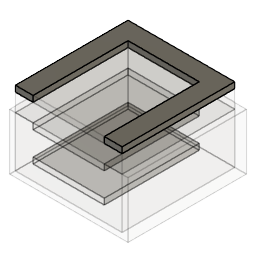
v3 (Autodesk Fusion 360 design; units mm, degrees)
part number: 2026-06-08-14-21-14-896
part number: 2026-06-08-14-24-47-444
part number: 2026-06-08-14-29-35-027
part number: 2026-06-08-14-30-01-795
part number: 2026-06-08-14-32-20-019
part number: 2026-06-08-14-37-08-306
part number: 2026-06-08-14-38-58-466
part number: 2026-06-08-14-44-18-946
part number: 2026-06-08-14-46-16-882
part number: 2026-06-09-12-46-36-713
Autodesk Fusion 360 part; units mm, degrees
sketch "Esquisse1" plane through (0, 0, 0) normal (0, 0, 1) x (1, 0, 0)
  line L0 (0, 0) -> (40, 0)
  line L1 (40, 0) -> (40, 40)
  line L2 (40, 40) -> (0, 40)
  line L3 (0, 40) -> (0, 0)
  dimension "d11" = 40
  dimension "d12" = 40
  constraint horizontal L0
  constraint vertical L1
  constraint horizontal L2
  constraint vertical L3
  constraint coincident L0.start L3.end
  measures "d11" distance of L0.start L0.end
  measures "d12" distance of L0.start L2.end
sketch "Esquisse1 (2)" plane through (0, 0, 2) normal (0, 0, 1) x (-1, 0, 0) in component "Shield"
  line L0 (0, -36) -> (0, 0)
  line L1 (0, 0) -> (-36, 0)
  line L2 (-36, 0) -> (-36, -36)
  line L3 (-36, -36) -> (0, -36)
  line L4 (0, -36) -> (-2, -36)
  line L5 (-2, -36) -> (-2, 4)
  line L6 (-2, 4) -> (0, 4)
  line L7 (0, 4) -> (0, -36)
  line L8 (0, -36) -> (-40, -36)
  line L9 (-40, -36) -> (-40, -34)
  line L10 (-40, -34) -> (0, -34)
  line L11 (0, -34) -> (0, -36)
  line L12 (-40, -36) -> (-38, -36)
  line L13 (-38, -36) -> (-38, 4)
  line L14 (-38, 4) -> (-40, 4)
  line L15 (-40, 4) -> (-40, -36)
  line L16 (-40, 4) -> (0, 4)
  line L17 (0, 4) -> (0, 2)
  line L18 (0, 2) -> (-40, 2)
  line L19 (-40, 2) -> (-40, 4)
  dimension "d15" = 2
  dimension "d16" = 40
  dimension "d17" = 40
  dimension "d18" = 2
  dimension "d19" = 2
  dimension "d20" = 40
  dimension "d21" = 40
  dimension "d22" = 2
  constraint horizontal L4
  constraint vertical L5
  constraint horizontal L6
  constraint vertical L7
  constraint coincident L0.start L3.end
  constraint horizontal L8
  constraint vertical L9
  constraint horizontal L10
  constraint vertical L11
  constraint horizontal L12
  constraint vertical L13
  constraint horizontal L14
  constraint vertical L15
  constraint horizontal L16
  constraint vertical L17
  constraint horizontal L18
  constraint vertical L19
  measures "d15" distance of L0.start L4.end
  measures "d16" distance of L0.start L6.end
  measures "d17" distance of L0.start L8.end
  measures "d18" distance of L0.start L10.end
  measures "d19" distance of L8.end L12.end
  measures "d20" distance of L8.end L14.end
  measures "d21" distance of L14.end L6.end
  measures "d22" distance of L14.end L18.end
sketch "Esquisse2" plane through (0, 0, 2) normal (0, 0, 1) x (-1, 0, 0) in component "Shield"
  line L0 (-36, -2) -> (-34, -2)
  line L1 (-34, -2) -> (-34, -34)
  line L2 (-34, -34) -> (-2, -34)
  line L3 (-2, -34) -> (-2, -2)
  line L4 (-2, -2) -> (0, -2)
  line L5 (0, -2) -> (0, 0)
  line L6 (0, 0) -> (-36, 0)
  line L7 (-36, 0) -> (-36, -2)
sketch "Esquisse1 (3)" plane through (0, 0, 6) normal (0, 0, 1) x (-1, 0, 0) in component "e*"
  line L0 (-36, 0) -> (-36, -2)
  line L1 (-36, -2) -> (-34, -2)
  line L2 (-34, -2) -> (-34, -34)
  line L3 (-34, -34) -> (-2, -34)
  line L4 (-2, -34) -> (-2, -2)
  line L5 (-2, -2) -> (0, -2)
  line L6 (0, -2) -> (0, 0)
  line L7 (0, 0) -> (-36, 0)
  line L8 (-8, -28) -> (-28, -28)
  line L9 (-28, -28) -> (-28, -3.2536)
  line L10 (-28, -3.2536) -> (-8, -3.2536)
  line L11 (-8, -3.2536) -> (-8, -28)
  dimension "d27" = 6
  dimension "d28" = 6
  dimension "d30" = 6
  constraint horizontal L8
  constraint vertical L9
  constraint horizontal L10
  constraint vertical L11
  measures "d27" distance of L4 L11
  measures "d28" distance of L2 L9
  measures "d30" distance of L3 L8
sketch "Esquisse1 (4)" plane through (0, 0, 16) normal (0, 0, 1) x (-1, 0, 0) in component "plaque_haut"
  line L0 (-2, 0) -> (-34, 0)
  line L1 (-34, 0) -> (-34, -34)
  line L2 (-34, -34) -> (-2, -34)
  line L3 (-2, -34) -> (-2, 0)
  line L4 (-6, -30) -> (-30, -30)
  line L5 (-30, -30) -> (-30, 0)
  line L6 (-30, 0) -> (-6, 0)
  line L7 (-6, 0) -> (-6, -30)
  dimension "d39" = 24
  dimension "d40" = 30
  constraint horizontal L4
  constraint vertical L5
  constraint horizontal L6
  constraint vertical L7
  measures "d39" distance of L4.start L4.end
  measures "d40" distance of L4.start L6.end
sketch "Esquisse1 (5)" plane through (0, 0, 18) normal (0, 0, 1) x (-1, 0, 0) in component "Mousse_haute"
  line L0 (0, -36) -> (0, -2)
  line L1 (0, -2) -> (-2, -2)
  line L2 (-2, -2) -> (-2, -34)
  line L3 (-2, -34) -> (-34, -34)
  line L4 (-34, -34) -> (-34, -2)
  line L5 (-34, -2) -> (-36, -2)
  line L6 (-36, -2) -> (-36, -36)
  line L7 (-36, -36) -> (0, -36)
  line L8 (0, -36) -> (-36, -36)
  line L9 (-36, -36) -> (-36, 0)
  line L10 (-36, 0) -> (0, 0)
  line L11 (0, 0) -> (0, -36)
  constraint horizontal L8
  constraint vertical L9
  constraint horizontal L10
  constraint vertical L11
  constraint coincident L0.start L7.end
sketch "Esquisse2 (2)" plane through (0, 0, 0) normal (0, 0, 1) x (1, 0, 0)
  line L0 (0, 0) -> (40, 0)
  line L1 (40, 0) -> (40, 40)
  line L2 (40, 40) -> (0, 40)
  line L3 (0, 40) -> (0, 0)
  dimension "d85" = 40
  dimension "d86" = 40
  constraint horizontal L0
  constraint vertical L1
  constraint horizontal L2
  constraint vertical L3
  constraint coincident L0.start L3.end
  measures "d85" distance of L0.start L0.end
  measures "d86" distance of L0.start L2.end
extrude "Extrusion4" add sketch "Esquisse2 (2)" along normal blind 2 makes body 1 in component "Shield"
sketch "Esquisse3" plane through (0, 0, 2) normal (0, 0, 1) x (-1, 0, 0)
  line L0 (0, -40) -> (0, 0)
  line L1 (0, 0) -> (-40, 0)
  line L2 (-40, 0) -> (-40, -40)
  line L3 (-40, -40) -> (0, -40)
  line L4 (0, -40) -> (-2, -40)
  line L5 (-2, -40) -> (-2, 0)
  line L6 (-2, 0) -> (0, 0)
  line L7 (0, 0) -> (0, -40)
  line L8 (0, -40) -> (-40, -40)
  line L9 (-40, -40) -> (-40, -38)
  line L10 (-40, -38) -> (0, -38)
  line L11 (0, -38) -> (0, -40)
  line L12 (-40, -40) -> (-38, -40)
  line L13 (-38, -40) -> (-38, 0)
  line L14 (-38, 0) -> (-40, 0)
  line L15 (-40, 0) -> (-40, -40)
  dimension "d89" = 2
  dimension "d90" = 40
  dimension "d91" = 40
  dimension "d92" = 2
  dimension "d93" = 2
  dimension "d94" = 40
  constraint horizontal L4
  constraint vertical L5
  constraint horizontal L6
  constraint vertical L7
  constraint coincident L0.start L3.end
  constraint horizontal L8
  constraint vertical L9
  constraint horizontal L10
  constraint vertical L11
  constraint horizontal L12
  constraint vertical L13
  constraint horizontal L14
  constraint vertical L15
  measures "d89" distance of L0.start L4.end
  measures "d90" distance of L0.start L0.end
  measures "d91" distance of L0.start L2.end
  measures "d92" distance of L0.start L10.end
  measures "d93" distance of L2.end L12.end
  measures "d94" distance of L2.end L1.end
extrude "Extrusion15" add sketch "Esquisse3" along normal blind 5 separate body contours L1 L5 L10 L13 makes body 2 in component "Support"
sketch "Esquisse1 (6)" plane through (0, 0, 7) normal (0, 0, 1) x (-1, 0, 0) in component "Plaque bas"
  line L0 (-38, -38) -> (-2, -38)
  line L1 (-2, -38) -> (-2, 0)
  line L2 (-2, 0) -> (-38, 0)
  line L3 (-38, 0) -> (-38, -38)
  line L4 (-8, 0) -> (-32, 0)
  line L5 (-32, 0) -> (-32, -32)
  line L6 (-32, -32) -> (-8, -32)
  line L7 (-8, -32) -> (-8, 0)
  dimension "d100" = 6
  dimension "d101" = 6
  dimension "d102" = 6
  constraint horizontal L4
  constraint vertical L5
  constraint horizontal L6
  constraint vertical L7
  constraint coincident L2 L4.start
  measures "d100" distance of L1 L7
  measures "d101" distance of L3 L5
  measures "d102" distance of L0 L6
extrude "Extrusion16" add sketch "Esquisse1 (6)" along normal blind 2 contours L0 L1 L2 L3 L5 L6 L7 bodies 2 in component "Support"
extrude "Extrusion5" add 1 faces at (16, 21.3333, 7) along direction (0, 0, 1) blind 2 separate body on bodies 2 makes body 3 in component "Plaque bas"
extrude "Extrusion17" add 1 faces at (36, 23.3333, 9) along direction (0, 0, 1) blind 8 on bodies 2 bodies 2 in component "Support"
extrude "Extrusion18" add 1 faces at (16, 21.3333, 9) along direction (0, 0, 1) blind 8 on bodies 3 bodies 2 in component "Support"
sketch "Esquisse2 (3)" plane through (0, 0, 17) normal (0, 0, 1) x (-1, 0, 0) in component "plaque_haut"
  line L0 (-2, 0) -> (-38, 0)
  line L1 (-38, 0) -> (-38, -38)
  line L2 (-38, -38) -> (-2, -38)
  line L3 (-2, -38) -> (-2, 0)
  line L4 (-8, 0) -> (-32, 0)
  line L5 (-32, 0) -> (-32, -32)
  line L6 (-32, -32) -> (-8, -32)
  line L7 (-8, -32) -> (-8, 0)
  point P0 (-32, 0)
  dimension "d111" = 6
  dimension "d112" = 6
  dimension "d113" = 6
  constraint horizontal L4
  constraint vertical L5
  constraint horizontal L6
  constraint vertical L7
  constraint coincident L4 P0
  measures "d111" distance of L2 L6
  measures "d112" distance of L1 L5
  measures "d113" distance of L3 L7
extrude "Extrusion5'" add sketch "Esquisse2 (3)" along normal blind 2 separate body contours L0 L4 L5 L6 L7 makes body 4 in component "plaque_haut"
extrude "Extrusion19" add 1 faces at (14, 12.6667, 17) along direction (0, 0, 1) blind 2 on bodies 2 bodies 2 in component "Support"
copy_body "CopierCollerCorps3" bodies 4 makes body 5 in component "Support"
combine "Combiner2" operation cut target body 2 tool bodies 5 in component "Support"
extrude "Extrusion2" add 1 faces at (16, 21.3333, 19) along direction (0, 0, 1) blind 6 separate body on bodies 4 makes body 6 in component "Mousse_haute"
extrude "Extrusion3" add 1 faces at (36, 23.3333, 19) along direction (0, 0, 1) blind 6 on bodies 2 bodies 6 in component "Mousse_haute"
extrude "Extrusion5''" add 1 faces at (13.3333, 13.3333, 2) along direction (0, 0, 1) blind 17 on bodies 1 bodies 1 in component "Shield"
copy_body "CopierCollerCorps1" bodies 3 makes body 7 in component "Shield"
copy_body "CopierCollerCorps2" bodies 4 7 makes body 8 makes body 9 in component "Shield"
copy_body "CopierCollerCorps3'" bodies 4 makes body 10 in component "Shield"
combine "Combiner1" operation cut target body 1 tool bodies 7 8 9 10 in component "Shield"
sketch "Esquisse1 (7)" plane through (0, 0, 25) normal (0, 0, 1) x (-1, 0, 0) in component "Support"
  line L0 (-2, 0) -> (-38, 0)
  line L1 (-38, 0) -> (-38, -38)
  line L2 (-38, -38) -> (-2, -38)
  line L3 (-2, -38) -> (-2, 0)
  line L4 (-8, 0) -> (-32, 0)
  line L5 (-32, 0) -> (-32, -32)
  line L6 (-32, -32) -> (-8, -32)
  line L7 (-8, -32) -> (-8, 0)
  dimension "d124" = 6
  dimension "d125" = 6
  dimension "d126" = 6
  constraint horizontal L4
  constraint vertical L5
  constraint horizontal L6
  constraint vertical L7
  constraint coincident L0 L4.start
  measures "d124" distance of L1 L5
  measures "d125" distance of L3 L7
  measures "d126" distance of L2 L6
extrude "Extrusion2'" add sketch "Esquisse1 (7)" along normal blind 2 separate body contours L0 L4 L5 L6 L7 makes body 11 in component "plateau_conducteur"
extrude "Extrusion1" add 1 faces at (14, 12.6667, 25) along direction (0, 0, 1) blind 2 separate body on bodies 6 makes body 12 in component "plateau_non_conducteur"
copy_body "CopierCollerCorps1'" bodies 11 makes body 13 in component "plateau_non_conducteur"
combine "Combiner1'" operation cut target body 12 tool bodies 13 in component "plateau_non_conducteur"
component "Shield" placed x (1, 0, 0) y (0, 1, 0) z (0, 0, 1) at (0, 0, 0)
component "Plaque bas" placed x (1, 0, 0) y (0, 1, 0) z (0, 0, 1) at (0, 0, 0)
component "Support" placed x (1, 0, 0) y (0, 1, 0) z (0, 0, 1) at (0, 0, 0)
component "Mousse_basse" placed x (1, 0, 0) y (0, 1, 0) z (0, 0, 1) at (0, 0, 0)
component "plaque_haut" placed x (1, 0, 0) y (0, 1, 0) z (0, 0, 1) at (0, 0, 0)
component "Mousse_haute" placed x (1, 0, 0) y (0, 1, 0) z (0, 0, 1) at (0, 0, 0)
component "plateau_conducteur" placed x (1, 0, 0) y (0, 1, 0) z (0, 0, 1) at (0, 0, 0)
component "plateau_non_conducteur" placed x (1, 0, 0) y (0, 1, 0) z (0, 0, 1) at (0, 0, 0)
component "e*" placed x (1, 0, 0) y (0, 1, 0) z (0, 0, 1) at (0, 0, 0) in component "Plaque bas"
equation "Deltax = 8 mm"
equation "Largeur_electrode = 8 mm"
equation "Longeur = 20 mm"
equation "epaisseur_mousse = 6 mm"
equation "Hauteur_support = 5 mm"
equation "deltad = 8 mm"
equation "Hauteur = epaisseur_mousse + epaisseur_electrode + deltad + Hauteur_support"
equation "Largeur = Deltax + 2 * Largeur_electrode + 2 * distance_bord_electrode + 2 * epaisseur_electrode"
equation "epaisseur_electrode = 2 mm"
equation "distance_bord_electrode = 6 mm"
equation "d11 = Largeur"
equation "d12 = Largeur"
equation "d15 = epaisseur_electrode"
equation "d16 = Largeur"
equation "d17 = Largeur"
equation "d18 = epaisseur_electrode"
equation "d19 = epaisseur_electrode"
equation "d20 = Largeur"
equation "d21 = Largeur"
equation "d22 = epaisseur_electrode"
equation "d27 = distance_bord_electrode"
equation "d28 = distance_bord_electrode"
equation "d30 = distance_bord_electrode"
equation "d39 = Largeur - 2 * distance_bord_electrode - 2 * epaisseur_electrode"
equation "d40 = Largeur - distance_bord_electrode - 2 * epaisseur_electrode"
equation "d85 = Largeur"
equation "d86 = Largeur"
equation "d87 = epaisseur_electrode"
equation "d89 = epaisseur_electrode"
equation "d90 = Largeur"
equation "d91 = Largeur"
equation "d92 = epaisseur_electrode"
equation "d93 = epaisseur_electrode"
equation "d94 = Largeur"
equation "d95 = Hauteur_support"
equation "d100 = distance_bord_electrode"
equation "d101 = distance_bord_electrode"
equation "d102 = distance_bord_electrode"
equation "d103 = epaisseur_electrode"
equation "d105 = epaisseur_electrode"
equation "d107 = deltad"
equation "d109 = deltad"
equation "d111 = distance_bord_electrode"
equation "d112 = distance_bord_electrode"
equation "d113 = distance_bord_electrode"
equation "d114 = epaisseur_electrode"
equation "d116 = epaisseur_electrode"
equation "d118 = epaisseur_mousse"
equation "d120 = epaisseur_mousse"
equation "d122 = deltad + 2 * epaisseur_electrode + Hauteur_support"
equation "d124 = distance_bord_electrode"
equation "d125 = distance_bord_electrode"
equation "d126 = distance_bord_electrode"
equation "d127 = epaisseur_electrode"
equation "d129 = epaisseur_electrode"
